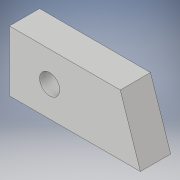
# Autodesk Inventor part: final orthograph
Saved by Autodesk Inventor 2017 (Build 210142000, 142)
## iProperties
Created: 2019-06-04
Part Number: final orthograph
Material: Generic
Document SubType Name: Modeling
Designer: qthuynh
Density: 1 g/cm^3
Appearance: Default
Author: qthuynh
Autodesk Inventor part; units mm, degrees
ref_plane "YZ Plane" through (0, 0, 0) normal (1, 0, 0) x (0, 1, 0)
ref_plane "XZ Plane" through (0, 0, 0) normal (0, 1, 0) x (-1, 0, 0)
ref_plane "XY Plane" through (0, 0, 0) normal (0, 0, 1) x (1, 0, 0)
sketch "Sketch1" plane through (0, 0, 0) normal (0, 0, 1) x (1, 0, 0)
  line L0 (0, 0) -> (82.55, 0)
  line L1 (0, 0) -> (0, 38.1)
  line L2 (0, 38.1) -> (69.85, 38.1)
  line L3 (69.85, 38.1) -> (82.55, 0)
  circle A0 centre (25.4, 19.05) radius 6.35
  dimension "d0" = 82.55
  dimension "d1" = 38.1
  dimension "d2" = 69.85
  dimension "d3" = 12.7
  dimension "d4" = 19.05
  dimension "d5" = 25.4
  constraints: 8 end point, 2 horizontal, 1 centre point, 1 vertical
  measures "d0" distance of L0.start L0.end
  measures "d1" distance of L0.start L1.end
  measures "d2" distance of L1.end L2.end
  measures "d3" diameter of A0
  measures "d4" distance from line of L2 A0.centre
  measures "d5" distance from line of L1 A0.centre
extrude "Extrusion1" add sketch "Sketch1" along normal blind 19.05
body "Solid1"
